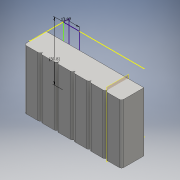
# Autodesk Inventor part: Battery
Saved by Autodesk Inventor 2016 (Build 200138000, 138)
## iProperties
Created: 2016-03-10
Part Number: Battery
Material: Generic
Document SubType Name: Modeling
Designer: Spencer
Density: 1 g/cm^3
Appearance: Default
Author: Spencer
Autodesk Inventor part; units mm, degrees
ref_plane "YZ Plane" through (0, 0, 0) normal (1, 0, 0) x (0, 1, 0)
ref_plane "XZ Plane" through (0, 0, 0) normal (0, 1, 0) x (-1, 0, 0)
ref_plane "XY Plane" through (0, 0, 0) normal (0, 0, 1) x (1, 0, 0)
sketch "Sketch1" plane through (0, 0, 0) normal (0, 1, 0) x (-1, 0, 0)
  line L0 (0, 0) -> (-69.85, 0)
  line L1 (-69.85, 0) -> (-69.85, -50.8)
  line L2 (-69.85, -50.8) -> (0, -50.8)
  line L3 (0, -50.8) -> (0, 0)
  dimension "d0" = 50.8
  dimension "d1" = 69.85
  constraints: 8 end point, 2 parallel, 1 horizontal, 1 perpendicular
  measures "d0" distance of L2.end L0.start
  measures "d1" distance of L0.start L0.end
extrude "Extrusion1" add sketch "Sketch1" along normal blind 28.575
sketch "Sketch2" plane through (0, 28.575, 0) normal (0, 1, 0) x (1, 0, 0)
  line L0 (0, 0) -> (69.85, 0) projected
  line L1 (13.97, 0) -> (13.97, 50.8)
  line L2 (69.85, 50.8) -> (0, 50.8) projected
  line L3 (27.94, 50.8) -> (27.94, 0)
  line L4 (55.88, 50.8) -> (55.88, 0)
  line L5 (41.91, 50.8) -> (41.91, 0)
  line L6 (0, 50.8) -> (0, 0) projected
  dimension "d4" = 13.97
  dimension "d5" = 13.97
  dimension "d6" = 13.97
  dimension "d7" = 13.97
  constraints: 8 end point, 8 point on line, 3 perpendicular, 1 vertical
  measures "d4" distance from line of L1.end L6
  measures "d5" distance from line of L3.start L1
  measures "d6" distance from line of L5.start L3
  measures "d7" distance from line of L4.start L5
sketch "Sketch3" plane through (0, 28.575, 0) normal (0, 1, 0) x (1, 0, 0)
  line L0 (69.85, 50.8) -> (0, 50.8) projected
  line L1 (0, 0) -> (69.85, 0) projected
  line L2 (0, 50.8) -> (13.97, 50.8)
  line L3 (13.97, 50.8) -> (13.97, 0)
  line L4 (13.97, 0) -> (0, 0)
  line L5 (0, 0) -> (0, 50.8)
  dimension "d8" = 50.8
  dimension "d9" = 13.97
  constraints: 8 end point, 2 parallel, 1 horizontal, 1 perpendicular, 1 point on line
  measures "d8" distance of L4.end L0.end
  measures "d9" distance from line of L1.start L3
extrude "Extrusion2" add sketch "Sketch2" along normal blind 5 contours L6 L2 L1 L0
sketch "Sketch4" plane through (0, 0, -50.8) normal (-1, 0, 0) x (0, 0, 1)
  line L0 (0, 0) -> (0, 33.575) projected
  line L1 (50.8, 0) -> (50.8, 33.575) projected
  line L2 (0, 33.575) -> (50.8, 33.575)
  line L3 (50.8, 33.575) -> (50.8, 28.5663)
  line L4 (50.8, 28.5663) -> (0, 28.5663)
  line L5 (0, 28.5663) -> (0, 33.575)
  constraints: 8 end point, 2 parallel, 1 horizontal, 1 perpendicular, 1 point on line
fillet "Fillet1" radius 2 2 edges at (0, 33.575, -25.4) (13.97, 33.575, -25.4)
sketch "Sketch5" plane through (0, 28.575, 0) normal (0, 1, 0) x (1, 0, 0)
  line L0 (13.97, 50.8) -> (27.94, 50.8)
  line L1 (27.94, 50.8) -> (27.94, 0)
  line L2 (27.94, 0) -> (13.97, 0)
  line L3 (13.97, 0) -> (13.97, 50.8)
  point P0 (0, 0)
  dimension "d13" = 13.97
  constraints: 8 end point, 2 parallel, 1 horizontal, 1 perpendicular
  measures "d13" distance of L1.end L2.end
extrude "Extrusion3" add sketch "Sketch5" along normal blind 5
fillet "Fillet2" radius 2 2 edges at (13.97, 33.575, -25.4) (27.94, 33.575, -25.4)
sketch "Sketch6" plane through (0, 28.575, 0) normal (0, 1, 0) x (1, 0, 0)
  line L0 (27.94, 50.8) -> (27.94, 0) projected
  line L1 (27.94, 50.8) -> (41.91, 50.8)
  line L2 (41.91, 50.8) -> (41.91, 0)
  line L3 (41.91, 0) -> (27.94, 0)
  line L4 (27.94, 0) -> (27.94, 50.8)
  point P0 (0, 0)
  dimension "d17" = 13.97
  constraints: 8 end point, 2 parallel, 1 horizontal, 1 perpendicular
  measures "d17" distance of L2.end L3.end
extrude "Extrusion4" add sketch "Sketch6" along normal blind 5
fillet "Fillet3" radius 2 2 edges at (27.94, 33.575, -25.4) (41.91, 33.575, -25.4)
sketch "Sketch7" plane through (0, 28.575, 0) normal (0, 1, 0) x (1, 0, 0)
  line L0 (41.91, 0) -> (41.91, 50.8) projected
  line L1 (41.91, 0) -> (69.85, 0) projected
  line L2 (41.91, 50.8) -> (55.88, 50.8)
  line L3 (55.88, 50.8) -> (55.88, 0)
  line L4 (55.88, 0) -> (41.91, 0)
  line L5 (41.91, 0) -> (41.91, 50.8)
  point P0 (0, 0)
  constraints: 8 end point, 2 parallel, 1 horizontal, 1 midpoint, 1 perpendicular
extrude "Extrusion5" add sketch "Sketch7" along normal blind 5
fillet "Fillet4" radius 2 2 edges at (41.91, 33.575, -25.4) (55.88, 33.575, -25.4)
sketch "Sketch8" plane through (0, 28.575, 0) normal (0, 1, 0) x (1, 0, 0)
  line L0 (55.88, 50.8) -> (55.88, 0) projected
  line L1 (55.88, 0) -> (69.85, 0) projected
  line L2 (55.88, 50.8) -> (69.85, 50.8)
  line L3 (69.85, 50.8) -> (69.85, 0)
  line L4 (69.85, 0) -> (55.88, 0)
  line L5 (55.88, 0) -> (55.88, 50.8)
  point P0 (0, 0)
  constraints: 8 end point, 2 parallel, 1 horizontal, 1 perpendicular
extrude "Extrusion6" add sketch "Sketch8" along normal blind 5
fillet "Fillet5" radius 2 2 edges at (55.88, 33.575, -25.4) (69.85, 33.575, -25.4)
sketch "Sketch9" plane through (0, 0, 0) normal (0, -1, 0) x (1, 0, 0)
  point P0 (0, 0)
sketch "Sketch10" plane through (0, 0, 0) normal (0, -1, 0) x (1, 0, 0)
  line L0 (69.85, -50.8) -> (0, -50.8) projected
  line L1 (0, 0) -> (13.97, 0)
  line L2 (13.97, 0) -> (13.97, -50.8)
  line L3 (13.97, -50.8) -> (0, -50.8)
  line L4 (0, -50.8) -> (0, 0)
  dimension "d27" = 13.97
  constraints: 8 end point, 2 parallel, 1 horizontal, 1 perpendicular, 1 point on line
  measures "d27" distance from line of L0.end L2
extrude "Extrusion7" add sketch "Sketch10" along normal blind 5
fillet "Fillet6" radius 2 2 edges at (0, -5, -25.4) (13.97, -5, -25.4)
sketch "Sketch11" plane through (0, 0, 0) normal (0, -1, 0) x (1, 0, 0)
  line L0 (13.97, 0) -> (13.97, -50.8) projected
  line L1 (27.94, -50.8) -> (25.94, -50.8) projected
  line L2 (13.97, 0) -> (27.94, 0)
  line L3 (27.94, 0) -> (27.94, -50.8)
  line L4 (27.94, -50.8) -> (13.97, -50.8)
  line L5 (13.97, -50.8) -> (13.97, 0)
  point P0 (0, 0)
  constraints: 8 end point, 2 parallel, 1 horizontal, 1 perpendicular
extrude "Extrusion8" add sketch "Sketch11" along normal blind 5
fillet "Fillet7" radius 2 2 edges at (13.97, -5, -25.4) (27.94, -5, -25.4)
sketch "Sketch12" plane through (0, 0, 0) normal (0, -1, 0) x (1, 0, 0)
  line L0 (27.94, 0) -> (27.94, -50.8) projected
  line L1 (41.91, 0) -> (41.91, -50.8) projected
  line L2 (27.94, 0) -> (41.91, 0)
  line L3 (41.91, 0) -> (41.91, -50.8)
  line L4 (41.91, -50.8) -> (27.94, -50.8)
  line L5 (27.94, -50.8) -> (27.94, 0)
  point P0 (0, 0)
  constraints: 8 end point, 2 parallel, 1 horizontal, 1 perpendicular
extrude "Extrusion9" add sketch "Sketch12" along normal blind 5
fillet "Fillet8" radius 2 2 edges at (27.94, -5, -25.4) (41.91, -5, -25.4)
sketch "Sketch13" plane through (0, 0, 0) normal (0, -1, 0) x (1, 0, 0)
  line L0 (41.91, -50.8) -> (41.91, 0) projected
  line L1 (69.85, -50.8) -> (41.91, -50.8) projected
  line L2 (41.91, 0) -> (55.88, 0)
  line L3 (55.88, 0) -> (55.88, -50.8)
  line L4 (55.88, -50.8) -> (41.91, -50.8)
  line L5 (41.91, -50.8) -> (41.91, 0)
  point P0 (0, 0)
  constraints: 8 end point, 2 parallel, 1 horizontal, 1 midpoint, 1 perpendicular
extrude "Extrusion10" add sketch "Sketch13" along normal blind 5
fillet "Fillet9" radius 2 2 edges at (55.88, -5, -25.4) (41.91, -5, -25.4)
sketch "Sketch14" plane through (0, 0, 0) normal (0, -1, 0) x (1, 0, 0)
  line L0 (53.88, 0) -> (55.88, 0) projected
  line L1 (69.85, -50.8) -> (55.88, -50.8) projected
  line L2 (55.88, 0) -> (69.85, 0)
  line L3 (69.85, 0) -> (69.85, -50.8)
  line L4 (69.85, -50.8) -> (55.88, -50.8)
  line L5 (55.88, -50.8) -> (55.88, 0)
  point P0 (0, 0)
  constraints: 8 end point, 2 parallel, 1 horizontal, 1 perpendicular
extrude "Extrusion11" add sketch "Sketch14" along normal blind 5
fillet "Fillet10" radius 2 2 edges at (55.88, -5, -25.4) (69.85, -5, -25.4)
sketch "Sketch15" plane through (2, 33.575, 0) normal (0, 0, 1) x (1, 0, 0)
  line L0 (-2, -2) -> (-2, -36.575) projected
  line L1 (-2, -19.2875) -> (67.85, -19.2875)
  line L2 (67.85, -36.575) -> (67.85, -2) projected
  line L3 (-2, -19.2875) -> (-2, 10.3755)
  line L4 (-2, 10.3755) -> (71.5202, 10.3755)
  line L5 (71.5202, 10.3755) -> (67.85, -19.2875)
  point P0 (-2, -33.575)
  constraints: 8 end point, 2 midpoint, 1 perpendicular, 1 point on line
extrude "Extrusion12" cut sketch "Sketch15" against normal through all
sketch "Sketch16" plane through (69.85, -3, 0) normal (1, 0, 0) x (0, 0, -1)
  line L0 (50.8, 17.2875) -> (0, 17.2875) projected
  line L1 (0, 0) -> (0, 17.2875) projected
  line L2 (50.8, 0) -> (0, 0) projected
  line L3 (50.8, 0) -> (50.8, 17.2875) projected
  point P0 (0, 3)
extrude "Extrusion13" add sketch "Sketch16" along normal blind 13.97
ref_plane "Work Plane1" through (69.85, -3, 0) normal (1, 0, 0) x (0, 0, -1)
mirror "Mirror1" about plane through (69.85, -3, 0) normal (1, 0, 0) of "Fillet10", "Extrusion11"
body "Solid1"
